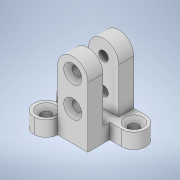
# Autodesk Inventor part: Крепление камеры к корпусу
Saved by Autodesk Inventor 2020 (Build 240168000, 168)
## iProperties
Created: 2021-04-13
Part Number: Крепление камеры к корпусу
Material: Типовые
Document SubType Name: Modeling
Designer: Антон
Density: 1 g/cm^3
Appearance: По умолчанию
Author: Антон
Autodesk Inventor part; units mm, degrees
note: some values were not read from the file. Chosen so that the rebuilt part matches the saved one: direction of "Отверстие1".
ref_plane "YZ Plane" through (0, 0, 0) normal (1, 0, 0) x (0, 1, 0)
sketch "Эскиз3" plane through (0, 0, 0) normal (0, 1, 0) x (-1, 0, 0)
  line L0 (0, 0) -> (10, 0)
  line L1 (10, 0) -> (10, -5)
  line L2 (10, -5) -> (0, -5)
  line L3 (0, -5) -> (0, 0)
  dimension "d6" = 10
  dimension "d7" = 5
  constraints: 8 end point, 2 parallel, 1 horizontal, 1 perpendicular
  measures "d6" distance of L1.end L2.end
  measures "d7" distance of L0.end L1.end
extrude "Выдавливание2" add sketch "Эскиз3" along normal blind 20
fillet "Сопряжение1" radius 5 2 edges at (0, 20, -2.5) (-10, 20, -2.5)
ref_plane "РабПлоскость1" through (0, 0, -7.6) normal (0, 0, -1) x (-1, 0, 0)
mirror "Зеркальное отражение1" about plane through (0, 0, -7.6) normal (0, 0, -1)
ref_plane "РабПлоскость2" through (0, 0, -12.9) normal (0, 0, -1) x (-1, 0, 0)
sketch "Эскиз5" plane through (-10, 0, 0) normal (0, 0, 1) x (1, 0, 0)
  arc A0 (10, 15) -> (0, 15) centre (5, 15) ccw projected
  line L0 (5, 15) -> (5, 5)
  dimension "d23" = 10
  constraints: 2 end point, 1 vertical
  measures "d23" distance of L0.start L0.end
hole "Отверстие1" at (-5, 15, 0) at (-5, 5, 0) direction (0, 0, -1) diameter 3.2 depth 12.9 countersink diameter 6 countersink angle 90
sketch "Эскиз6" plane through (-10, 0, -15.2) normal (0, 0, 1) x (1, 0, 0)
  circle A0 centre (5, 15) radius 1.6 projected
  circle A1 centre (5, 5) radius 1.6 projected
  line L0 (6.6166, 17.8) -> (8.2332, 15)
  line L1 (8.2332, 15) -> (6.6166, 12.2)
  line L2 (6.6166, 12.2) -> (3.3834, 12.2)
  line L3 (3.3834, 12.2) -> (1.7668, 15)
  line L4 (1.7668, 15) -> (3.3834, 17.8)
  line L5 (3.3834, 17.8) -> (6.6166, 17.8)
  line L6 (6.6166, 7.8) -> (8.2332, 5)
  line L7 (8.2332, 5) -> (6.6166, 2.2)
  line L8 (6.6166, 2.2) -> (3.3834, 2.2)
  line L9 (3.3834, 2.2) -> (1.7668, 5)
  line L10 (1.7668, 5) -> (3.3834, 7.8)
  line L11 (3.3834, 7.8) -> (6.6166, 7.8)
  point P0 (10, 0)
  dimension "d24" = 5.6
  dimension "d25" = 5.6
  constraints: 24 end point, 2 coincident, 26 other
  measures "d24" distance between parallel lines of L2 L5
  measures "d25" distance between parallel lines of L8 L11
extrude "Выдавливание3" cut sketch "Эскиз6" along normal up to surface (2.3 mm away) contours A0 | A1 | L0 L1 L2 L3 L4 L5 | L6 L7 L8 L9 L10 L11
sketch "Эскиз9" plane through (-10, 0, -15.2) normal (0, -1, 0) x (1, 0, 0)
  line L0 (0, 5) -> (0, 0) projected
  line L1 (10, 15.2) -> (0, 15.2)
  line L2 (0, 15.2) -> (0, 0)
  line L3 (0, 0) -> (10, 0)
  line L4 (10, 0) -> (10, 15.2)
  constraints: 8 end point, 2 parallel, 1 horizontal, 1 perpendicular
extrude "Выдавливание5" add sketch "Эскиз9" along normal blind 5
sketch "Эскиз11" plane through (-10, -5, -15.2) normal (0, -1, 0) x (1, 0, 0)
  line L0 (0, 15.2) -> (0, 0) projected
  line L1 (0, 0) -> (10, 0) projected
  line L2 (10, 0) -> (10, 15.2) projected
  line L3 (10, 15.2) -> (0, 15.2) projected
  line L4 (10, 0) -> (18, 0)
  line L5 (18, 0) -> (18, 8)
  line L6 (18, 8) -> (10, 8)
  line L7 (10, 8) -> (10, 0)
  line L8 (0, 0) -> (0, 2)
  line L9 (0, 5) -> (0, 0) projected
  line L10 (0, 2) -> (-8, 2)
  line L11 (-8, 2) -> (-8, 10)
  line L12 (-8, 10) -> (0, 10)
  line L13 (0, 10) -> (0, 2)
  line L14 (0, 10) -> (0, 11)
  line L15 (0, 10.2) -> (0, 15.2) projected
  line L16 (0, 11) -> (-8, 11)
  line L17 (-8, 11) -> (-8, 19)
  line L18 (-8, 19) -> (0, 19)
  line L19 (0, 19) -> (0, 11)
  point P0 (0, 2)
  dimension "d75" = 8
  dimension "d76" = 8
  dimension "d77" = 2
  dimension "d78" = 8
  dimension "d79" = 8
  dimension "d80" = 1
  dimension "d81" = 8
  dimension "d82" = 8
  constraints: 28 end point, 6 parallel, 3 horizontal, 3 perpendicular, 2 point on line
  measures "d75" distance of L6.end L5.end
  measures "d76" distance of L5.end L4.end
  measures "d77" distance of L0.end L8.end
  measures "d78" distance of L11.end L12.end
  measures "d79" distance of L10.end L11.end
  measures "d80" distance of L12.end L14.end
  measures "d81" distance of L17.end L18.end
  measures "d82" distance of L16.end L17.end
extrude "Выдавливание6" add sketch "Эскиз11" against normal blind 5 contours L0 L16 L17 L18 L19 | L6 L5 L4 L2 | L0 L10 L11 L12
sketch "Эскиз12" plane through (-10, 0, -15.2) normal (0, 1, 0) x (1, 0, 0)
  line L0 (10, -10.2) -> (0, -10.2) projected
  line L1 (10, -8) -> (10, -10.2) projected
  line L2 (10, -8) -> (18, -8) projected
  line L3 (18, -8) -> (18, 0) projected
  line L4 (18, 0) -> (10, 0) projected
  line L5 (10, -5) -> (10, 0) projected
  line L6 (10, -5) -> (0, -5) projected
  line L7 (0, -2) -> (0, -5) projected
  line L8 (0, -2) -> (-8, -2) projected
  line L9 (-8, -2) -> (-8, -10) projected
  line L10 (-8, -10) -> (0, -10) projected
  line L11 (0, -10.2) -> (0, -10) projected
  line L12 (0, -11) -> (-8, -11) projected
  line L13 (-8, -11) -> (-8, -19) projected
  line L14 (-8, -19) -> (0, -19) projected
  line L15 (0, -19) -> (0, -15.2) projected
  line L16 (0, -11) -> (0, -15.2) projected
  line L17 (0, -2) -> (-8, -2) projected
  line L18 (-4, -2) -> (-4, -10)
  line L19 (0, -11) -> (-8, -11) projected
  line L20 (-4, -11) -> (-4, -19)
  line L21 (18, 0) -> (10, 0) projected
  line L22 (14, 0) -> (14, -8)
  point P0 (10, -15.2)
  point P1 (14, -4)
  point P2 (-4, -6)
  point P3 (-4, -15)
  constraints: 9 midpoint, 6 end point
hole "Отверстие4" at (-14, 0, -9.2) at (4, 0, -11.2) at (-14, 0, -0.2) direction (0, -1, 0) diameter 3.2 end through all countersink diameter 6 countersink angle 90
fillet "Сопряжение2" radius 4 7 edges at (8, -2.5, -15.2) (8, -2.5, -7.2) (-18, -2.5, -13.2) (-18, -2.5, -5.2) (-18, -2.5, -4.2) (-18, -2.5, 3.8) (-10, -2.5, 3.8)
equation "\"d25\" = d24"
